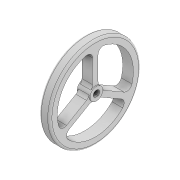
# Autodesk Inventor part: rear wheel 86mm
Saved by Autodesk Inventor 2022 (Build 260153000, 153)
## iProperties
Created: 2024-06-07
Part Number: rear wheel 86mm
Material: Generic
Document SubType Name: Modeling
Designer: david
Density: 1 g/cm^3
Appearance: Default
Author: david
Autodesk Inventor part; units mm, degrees
ref_plane "YZ Plane" through (0, 0, 0) normal (1, 0, 0) x (0, 1, 0)
ref_plane "XZ Plane" through (0, 0, 0) normal (0, 1, 0) x (-1, 0, 0)
ref_plane "XY Plane" through (0, 0, 0) normal (0, 0, 1) x (1, 0, 0)
sketch "Sketch1" plane through (0, 0, 0) normal (1, 0, 0) x (0, 1, 0)
  circle A0 centre (0, 0) radius 42.75
  dimension "d0" = 85.5
  constraints: 1 centre point, 1 coincident
  measures "d0" diameter of A0
extrude "Extrusion1" add sketch "Sketch1" along normal mid plane 10
fillet "Fillet1" radius 2 2 edges at (5, -42.75, 0) (-5, -42.75, 0)
sketch "Sketch2" plane through (0, 0, 0) normal (1, 0, 0) x (0, 1, 0)
  circle A0 centre (0, 0) radius 6
  dimension "d9" = 12
  constraints: 1 centre point, 1 coincident
  measures "d9" diameter of A0
extrude "Extrusion2" add sketch "Sketch2" along normal mid plane 12
sketch "Sketch3" plane through (-6, 0, 0) normal (1, 0, 0) x (0, 1, 0)
  arc A0 (-2.5, -1.6583) -> (-2.5, 1.6583) centre (0, 0) ccw
  line L0 (-2.5, -1.6583) -> (-2.5, 1.6583)
  dimension "d12" = 3
  dimension "d13" = 2.5
  constraints: 2 end point, 2 point on circle, 1 centre point, 1 coincident, 1 vertical
  measures "d12" radius of A0
  measures "d13" distance from line of L0 point (0, 0)
extrude "Extrusion3" cut sketch "Sketch3" along normal through all
sketch "Sketch4" plane through (5, 0, 0) normal (1, 0, 0) x (0, 0, -1)
  arc A0 (1.6583, -2.5) -> (-1.6583, -2.5) centre (0, 0) ccw projected
  circle A1 centre (0, 0) radius 35.75
  circle A2 centre (0, 0) radius 6 projected
  circle A3 centre (0, 0) radius 40.75 projected
  line L0 (2.5, 35.6625) -> (2.5, 0)
  line L1 (2.5, 0) -> (-2.5, 0)
  line L2 (-2.5, 0) -> (-2.5, 35.6625)
  line L3 (1.25, -2.1651) -> (-29.6346, -19.9963)
  line L4 (-32.1346, -15.6662) -> (-1.25, 2.1651)
  line L5 (1.25, 2.1651) -> (32.1346, -15.6662)
  line L6 (29.6346, -19.9963) -> (-1.25, -2.1651)
  line L7 (-1.6583, -2.5) -> (1.6583, -2.5) projected
  arc A4 (1.6583, -2.5) -> (-1.6583, -2.5) centre (0, 0) ccw projected
  point P0 (3.4736, -4.8922)
  point P1 (-3.4736, -4.8922)
  point P2 (5.9736, -0.5621)
  point P3 (2.5, 5.4544)
  point P4 (-5.9736, -0.5621)
  point P5 (-2.5, 5.4544)
  dimension "d17" = 71.5
  dimension "d18" = 5
  dimension "d21" = 360
  constraints: 14 end point, 2 coincident, 2 point on circle, 1 centre point, 1 horizontal, 1 midpoint, 1 parallel, 1 vertical, 19 other
  measures "d17" diameter of A1
  measures "d18" distance between parallel lines of L2 L0
extrude "Extrusion4" cut sketch "Sketch4" against normal through all contours A2 L0 A1 L5 | L6 A1 L3 A2 | A2 L4 A1 L2
fillet "Fillet2" radius 5 12 edges at (0, -19.9963, -29.6346) (0, -15.6662, -32.1346) (0, 35.6625, -2.5) (0, 35.6625, 2.5) (0, 5.4544, -2.5) (0, -0.5621, -5.9736) (0, 5.4544, 2.5) (0, -0.5621, 5.9736) (0, -15.6662, 32.1346) (0, -19.9963, 29.6346) (0, -4.8922, 3.4736) (0, -4.8922, -3.4736)
body "Solid1"
